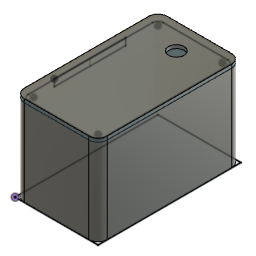
Button Case (Autodesk Fusion 360 design; units mm, degrees)
Autodesk Fusion 360 part; units mm, degrees
sketch "Base" plane through (0, 0, 0) normal (0, 1, 0) x (1, 0, 0) in component "Top"
  line L0 (0, 0) -> (36, 0)
  line L1 (36, 0) -> (36, 62)
  line L2 (36, 62) -> (0, 62)
  line L3 (0, 62) -> (0, 0)
  dimension "d6" = 36
  dimension "d7" = 62
  constraint horizontal L0
  constraint vertical L1
  constraint horizontal L2
  constraint vertical L3
  constraint coincident L0.start L3.end
  measures "d6" distance of L0.start L0.end
  measures "d7" distance of L0.start L2.end
extrude "Extrude1" add sketch "Base" along normal blind 37.5 makes body 1 in component "Top"
fillet "Fillet1" radius 4 4 edges at (36, 18.75, 0) (0, 18.75, 0) (36, 18.75, -62) (0, 18.75, -62) on bodies 1 in component "Top"
shell "Shell1" thickness 1.5 removed faces 1 at (12, 37.5, -22) on bodies 1 in component "Top"
sketch "Knob" plane through (1.5, 0, 0) normal (1, 0, 0) x (0, 0, -1) in component "Top"
  line L0 (58, 1.5) -> (58, 37.5)
  line L1 (58, 37.5) -> (4, 37.5)
  line L2 (4, 37.5) -> (4, 1.5)
  line L3 (4, 1.5) -> (58, 1.5)
  line L4 (15.5, 37.5) -> (46.5, 37.5)
  line L5 (46.5, 37.5) -> (46.5, 34.5)
  line L6 (46.5, 34.5) -> (15.5, 34.5)
  line L7 (15.5, 34.5) -> (15.5, 37.5)
  line L8 (31, 37.5) -> (31, 34.5) construction
  dimension "d12" = 31
  dimension "d13" = 3
  constraint horizontal L4
  constraint vertical L5
  constraint horizontal L6
  constraint vertical L7
  constraint coincident L1 L4.start
  constraint midpoint L1 L8.start
  constraint midpoint L6 L8.end
  constraint vertical L8
  measures "d12" distance of L5.end L6.end
  measures "d13" distance of L4.end L5.end
extrude "Extrude2" add sketch "Knob" along normal blind 6 draft -45 contours L1 L4 L5 L6 L7 bodies 1 in component "Top"
ref_plane "WorkPlane2" through (18, 18.75, -31) normal (-1, 0, 0) x (0, 0, 1) in component "Top"
mirror "Mirror1" about plane through (18, 18.75, -31) normal (-1, 0, 0) of "Extrude2" in component "Top"
sketch "Top" plane through (0, 37.5, 0) normal (0, 1, 0) x (-1, 0, 0) in component "Base"
  line L0 (-36, -4) -> (-36, -58)
  arc A0 (-36, -58) -> (-32, -62) centre (-32, -58) ccw
  line L1 (-32, -62) -> (-4, -62)
  arc A1 (-4, -62) -> (0, -58) centre (-4, -58) ccw
  line L2 (0, -58) -> (0, -4)
  arc A2 (0, -4) -> (-4, 0) centre (-4, -4) ccw
  line L3 (-4, 0) -> (-32, 0)
  arc A3 (-32, 0) -> (-36, -4) centre (-32, -4) ccw
  line L4 (-34.5, -15.5) -> (-34.5, -4)
  arc A4 (-32, -1.5) -> (-34.5, -4) centre (-32, -4) ccw
  line L5 (-32, -1.5) -> (-4, -1.5)
  arc A5 (-1.5, -4) -> (-4, -1.5) centre (-4, -4) ccw
  line L6 (-1.5, -4) -> (-1.5, -15.5)
  line L7 (-1.5, -15.5) -> (-1.5, -46.5)
  line L8 (-1.5, -46.5) -> (-1.5, -58)
  arc A6 (-4, -60.5) -> (-1.5, -58) centre (-4, -58) ccw
  line L9 (-4, -60.5) -> (-32, -60.5)
  arc A7 (-34.5, -58) -> (-32, -60.5) centre (-32, -58) ccw
  line L10 (-34.5, -58) -> (-34.5, -46.5)
  line L11 (-34.5, -46.5) -> (-34.5, -15.5)
extrude "Extrude1'" add sketch "Top" along normal blind 1.5 separate body contours L0 A0 L1 A1 L2 A2 L3 A3 | L4 A4 L5 A5 L6 L7 L8 A6 L9 A7 L10 L11 makes body 2 in component "Base"
sketch "Lip" plane through (0, 37.5, 0) normal (0, -1, 0) x (1, 0, 0) in component "Base"
  arc A0 (36, -4) -> (32, 0) centre (32, -4) ccw
  line L0 (32, 0) -> (4, 0)
  arc A1 (4, 0) -> (0, -4) centre (4, -4) ccw
  line L1 (0, -4) -> (0, -58)
  arc A2 (0, -58) -> (4, -62) centre (4, -58) ccw
  line L2 (4, -62) -> (32, -62)
  arc A3 (32, -62) -> (36, -58) centre (32, -58) ccw
  line L3 (36, -58) -> (36, -4)
  line L4 (34.3, -58) -> (34.3, -4)
  arc A4 (34.3, -4) -> (32, -1.7) centre (32, -4) ccw
  line L5 (32, -1.7) -> (4, -1.7)
  arc A5 (4, -1.7) -> (1.7, -4) centre (4, -4) ccw
  line L6 (1.7, -4) -> (1.7, -58)
  arc A6 (1.7, -58) -> (4, -60.3) centre (4, -58) ccw
  line L7 (4, -60.3) -> (32, -60.3)
  arc A7 (32, -60.3) -> (34.3, -58) centre (32, -58) ccw
  dimension "d19" = 1.7
extrude "Extrude2'" add sketch "Lip" along normal blind 3 contours L4 A4 L5 A5 L6 A6 L7 A7 bodies 2 in component "Base"
extrude "Extrude3" cut sketch "Knob" along normal blind 3 draft -45 from surface at 0.2 contours L1 L4 L5 L6 L7 bodies 2 in component "Base"
mirror "Mirror1'" about plane through (18, 18.75, -31) normal (-1, 0, 0) of "Extrude3" in component "Base"
shell "Shell1'" thickness 1.5 removed faces 1 at (23.4333, 34.5, -36.1667) on bodies 2 in component "Base"
chamfer "Chamfer1" distance 0.6 angle 45 2 edges at (1.7, 34.5, -31) (34.3, 34.5, -31) on bodies 2 in component "Base"
sketch "Sketch3" plane through (0, 39, 0) normal (0, 1, 0) x (-1, 0, 0)
  arc A0 (-32, 0) -> (-36, -4) centre (-32, -4) ccw
  line L0 (-36, -4) -> (-36, -58)
  arc A1 (-36, -58) -> (-32, -62) centre (-32, -58) ccw
  line L1 (-32, -62) -> (-4, -62)
  arc A2 (-4, -62) -> (0, -58) centre (-4, -58) ccw
  line L2 (0, -58) -> (0, -4)
  arc A3 (0, -4) -> (-4, 0) centre (-4, -4) ccw
  line L3 (-4, 0) -> (-32, 0)
  circle A4 centre (-19, -51) radius 3.35
  dimension "d55" = 6.7
  measures "d55" diameter of A4
extrude "Extrude6" cut sketch "Sketch3" along normal blind 0 and the other way blind 2 contours A4 bodies 2 in component "Base"
sketch "PCB Mount" plane through (0, 25, 0) normal (0, -1, 0) x (1, 0, 0) in component "Base"
  arc A0 (90, -4) -> (86, 0) centre (86, -4) ccw construction
  arc A1 (0, -46) -> (4, -50) centre (4, -46) ccw construction
  line L0 (88.8284, -1.1716) -> (1.1716, -48.8284) construction
  line L1 (67.5, -37.5) -> (22.5, -37.5)
  line L2 (22.5, -37.5) -> (22.5, -12.5)
  line L3 (22.5, -12.5) -> (67.5, -12.5)
  line L4 (67.5, -12.5) -> (67.5, -37.5)
  line L5 (67.5, -37.5) -> (22.5, -12.5) construction
  line L6 (22.5, -37.5) -> (67.5, -12.5) construction
  point P0 (45, -25)
  dimension "d33" = 18
  dimension "d34" = 31
  constraint midpoint A0 L0.start
  constraint midpoint A1 L0.end
  constraint perpendicular L1 L2
  constraint parallel L1 L3
  constraint parallel L2 L4
  constraint horizontal L1
  constraint coincident L5 P0
  constraint coincident L6 P0
  constraint midpoint L0 P0
extrude "Extrude5" [suppressed] in component "Base"
sketch "Right Holes" plane through (90, 0, 0) normal (1, 0, 0) x (0, 0, -1) in component "Top"
  line L0 (46, 25) -> (4, 25)
  line L1 (4, 25) -> (4, 0)
  line L2 (4, 0) -> (46, 0)
  line L3 (46, 0) -> (46, 25)
  circle A0 centre (25, 12.5) radius 3
  line L4 (0, 25) -> (0, 0)
  line L5 (0, 0) -> (50, 0)
  dimension "d41" = 6
  dimension "d42" = 31
  dimension "d43" = 18.75
  measures "d41" diameter of A0
extrude "Extrude3'" [suppressed] in component "Top"
sketch "Top Holes" plane through (0, 0, 0) normal (0, 1, 0) x (1, 0, 0) in component "Top"
  circle A0 centre (15, 30) radius 3
  circle A1 centre (75, 20) radius 3
  line L0 (0, 50) -> (0, 0)
  line L1 (90, 50) -> (0, 50)
  line L2 (0, 0) -> (90, 0)
  line L3 (90, 0) -> (90, 50)
  dimension "d46" = 6
  dimension "d47" = 6
  dimension "d48" = 15
  dimension "d49" = 20
  dimension "d50" = 20
  dimension "d51" = 15
  measures "d46" diameter of A0
  measures "d47" diameter of A1
  measures "d48" distance of A0.centre L0
  measures "d49" distance of A0.centre L1
  measures "d50" distance of A1.centre L2
  measures "d51" distance of A1.centre L3
extrude "Extrude4" [suppressed] in component "Top"
component "Enclosure" placed x (1, 0, 0) y (0, 1, 0) z (0, 0, 1) at (0, 0, 0)
component "Top" placed x (1, 0, 0) y (0, 1, 0) z (0, 0, 1) at (0, 0, 0) in component "Enclosure"
component "Base" placed x (1, 0, 0) y (0, 1, 0) z (0, 0, 1) at (0, 0, 0) in component "Enclosure"
equation "Width = 62 mm"
equation "length = 36 mm"
equation "heigth = 37.5 mm"
equation "shell = 1.5 mm"
equation "gap = 0.2 mm"
equation "d6 = length"
equation "d7 = Width"
equation "d8 = heigth"
equation "d11 = shell"
equation "d12 = Width / 2"
equation "d13 = shell * 2"
equation "d17 = shell"
equation "d19 = shell + gap"
equation "d20 = shell * 2"
equation "d23 = shell * 2"
equation "d26 = shell"
equation "d33 = length / 2"
equation "d34 = Width / 2"
equation "d42 = Width / 2"
equation "d43 = heigth / 2"
